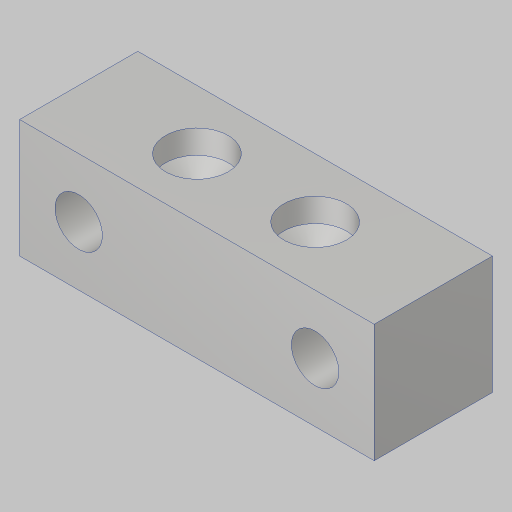
# Autodesk Inventor part: CL7-GB-004
Saved by Autodesk Inventor 2023.5 (Build 275446000, 446)
## iProperties
Created: 2025-03-18
Part Number: CL7-GB-004
Material: Aluminum 6061
Document SubType Name: Modeling
Designer: slick
Density: 2.7 g/cm^3
Appearance: Aluminum - Flat
Author: slick
Autodesk Inventor part; units mm, degrees
ref_plane "YZ Plane" through (0, 0, 0) normal (1, 0, 0) x (0, 1, 0)
ref_plane "XZ Plane" through (0, 0, 0) normal (0, 1, 0) x (-1, 0, 0)
ref_plane "XY Plane" through (0, 0, 0) normal (0, 0, 1) x (1, 0, 0)
sketch "Sketch1" plane through (0, 0, 0) normal (0, 0, 1) x (1, 0, 0)
  line L0 (19.05, -6.35) -> (-19.05, -6.35)
  line L1 (-19.05, -6.35) -> (-19.05, 6.35)
  line L2 (-19.05, 6.35) -> (19.05, 6.35)
  line L3 (19.05, 6.35) -> (19.05, -6.35)
  line L4 (19.05, -6.35) -> (-19.05, 6.35) construction
  line L5 (-19.05, -6.35) -> (19.05, 6.35) construction
  point P0 (0, 0)
  dimension "d0" = 38.1
  dimension "d1" = 12.7
  constraints: 12 end point, 2 midpoint, 2 parallel, 1 horizontal, 1 perpendicular
  measures "d0" distance of L1.end L2.end
  measures "d1" distance of L0.end L1.end
extrude "Extrusion1" add sketch "Sketch1" along normal blind 12.7
sketch "Sketch2" plane through (-19.05, 6.35, 0) normal (0, 1, 0) x (1, 0, 0)
  line L0 (0, 0) -> (0, -12.7) construction
  line L1 (12.7, -6.35) -> (25.4, -6.35) construction
  line L2 (38.1, 0) -> (0, 0) construction
  line L3 (38.1, -12.7) -> (0, -12.7) construction
  point P0 (19.05, 0)
  point P1 (0, -6.35)
  point P2 (19.05, -6.35)
  point P3 (19.05, 0)
  point P4 (19.05, 0)
  dimension "d4" = 12.7
  dimension "d20" = 6.35
  constraints: 4 midpoint, 2 end point, 2 vertical alignment, 1 horizontal alignment
  measures "d4" distance of L1.start L1.end
  measures "d20" distance between parallel lines of L3 L1
sketch "Sketch3" plane through (0, 0, 12.7) normal (0, 0, 1) x (1, 0, 0)
  line L0 (-12.7, 0) -> (12.7, 0) construction
  line L1 (-19.05, 6.35) -> (-19.05, -6.35) construction
  line L2 (19.05, 6.35) -> (-19.05, 6.35) construction
  point P0 (0, 0)
  point P1 (-19.05, 0)
  point P2 (0, 0)
  point P3 (0, 6.35)
  dimension "d12" = 25.4
  constraints: 3 midpoint, 2 end point, 1 horizontal, 1 horizontal alignment, 1 vertical alignment
  measures "d12" distance of L0.start L0.end
hole "Hole2" at (-12.7, 0, 12.7) at (12.7, 0, 12.7) direction (0, 0, -1) diameter 5.1054 end through all clearance for "Flat Head Machine Screw (82)" size "#10" standard "Ansi Unified Screw Threads"
hole "Hole3" at (-6.35, 6.35, 6.35) at (6.35, 6.35, 6.35) direction (0, -1, 0) diameter 6.7564 depth 2.54 tip angle 118 clearance for "Flat Head Machine Screw (82)" size "1/4" standard "Ansi Unified Screw Threads"
body "Solid1"
